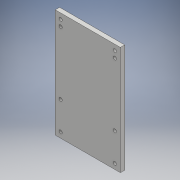
# Autodesk Inventor part: BaseRB
Saved by Autodesk Inventor 2017 SP1 (Build 210196100, 196)
## iProperties
Part Number: BaseRB
Material: Genérico
Document SubType Name: Modeling
Designer: Juan
Density: 1 g/cm^3
Appearance: Valor por defecto
Author: Juan
Autodesk Inventor part; units mm, degrees
ref_plane "YZ Plane" through (0, 0, 0) normal (1, 0, 0) x (0, 1, 0)
ref_plane "XZ Plane" through (0, 0, 0) normal (0, 1, 0) x (-1, 0, 0)
sketch "Boceto1" plane through (0, 0, 0) normal (0, 1, 0) x (-1, 0, 0)
  line L0 (60, 100) -> (60, 0)
  line L1 (60, 0) -> (0, 0)
  line L2 (0, 0) -> (0, 100)
  line L3 (0, 100) -> (60, 100)
  dimension "d0" = 100
  dimension "d1" = 60
  dimension "d2" = 100
  constraints: 8 end point, 2 perpendicular, 1 coincident, 1 vertical
  measures "d0" distance of L0.start L0.end
  measures "d1" distance of L0.end L1.end
  measures "d2" distance of L1.end L2.end
extrude "Extrusión1" add sketch "Boceto1" along normal blind 4
ref_plane "Plano de trabajo1" through (0, 2, 0) normal (0, 1, 0) x (1, 0, 0)
sketch "Boceto2" plane through (0, 4, 0) normal (0, 1, 0) x (1, 0, 0)
  line L0 (-60, -100) -> (0, -100) construction
  line L1 (-60, -100) -> (-60, -95) construction
  line L2 (-60, 0) -> (-60, -100) construction
  line L3 (-60, -95) -> (-55, -95) construction
  line L4 (-55, -95) -> (-55, -100) construction
  line L5 (0, -95) -> (-5, -95) construction
  line L6 (-5, -95) -> (-5, -100) construction
  line L7 (-60, 0) -> (-60, -5) construction
  line L8 (-60, -5) -> (-55, -5) construction
  line L9 (-55, -5) -> (-55, 0) construction
  line L10 (0, 0) -> (-60, 0) construction
  line L11 (-5, 0) -> (-5, -5) construction
  line L12 (-5, -5) -> (0, -5) construction
  dimension "d5" = 5
  dimension "d6" = 5
  dimension "d7" = 5
  dimension "d8" = 5
  constraints: 20 end point, 9 point on line, 5 perpendicular, 1 vertical
  measures "d5" distance of L0.start L1.end
  measures "d6" distance of L1.end L3.end
  measures "d7" distance of L5.start L5.end
  measures "d8" distance of L2.start L7.end
hole "Agujero1" at (-55.0115, 4, 95.0136) direction (0, -1, 0) diameter 3 depth 5 tip angle 118
hole "Agujero2" at (-4.9994, 4, 95.0021) direction (0, -1, 0) diameter 3 depth 5 tip angle 118
hole "Agujero3" at (-55.0247, 4, 5.111) direction (0, -1, 0) diameter 3 depth 5 tip angle 118
hole "Agujero4" at (-5.0158, 4, 5.0059) direction (0, -1, 0) diameter 3 depth 5 tip angle 118
sketch "Boceto3" plane through (0, 4, 0) normal (0, 1, 0) x (1, 0, 0)
  circle A0 centre (-55.0115, -95.0136) radius 1.5 construction
  line L0 (-55.0115, -95.0136) -> (-55.0115, -89.0136) construction
  circle A1 centre (-4.9994, -95.0021) radius 1.5 construction
  line L1 (-4.9994, -95.0021) -> (-4.9994, -89.0021) construction
  circle A2 centre (-55.0247, -5.111) radius 1.5 construction
  circle A3 centre (-5.0158, -5.0059) radius 1.5 construction
  line L2 (-55.0115, -89.0136) -> (-55.0115, -31.0136) construction
  line L3 (-4.9994, -89.0021) -> (-4.9994, -31.0021) construction
  point P0 (0, 0)
  dimension "d45" = 6
  dimension "d46" = 6
  dimension "d49" = 58
  dimension "d50" = 58
  constraints: 8 end point, 4 vertical
  measures "d45" distance of L0.start L0.end
  measures "d46" distance of L1.start L1.end
  measures "d49" distance of L0.end L2.end
  measures "d50" distance of L1.end L3.end
hole "Agujero5" at (-55.062, 4, 89.0456) direction (0, -1, 0) diameter 3 depth 5 tip angle 118
hole "Agujero6" at (-4.9884, 4, 89.0265) direction (0, -1, 0) diameter 3 depth 5 tip angle 118
hole "Agujero7" at (-55.0837, 4, 31.0333) direction (0, -1, 0) diameter 3 depth 5 tip angle 118
hole "Agujero8" at (-5.0141, 4, 30.9969) direction (0, -1, 0) diameter 3 depth 5 tip angle 118
